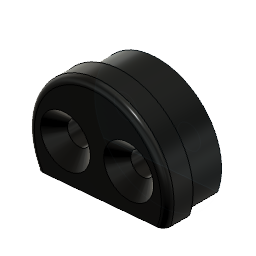
012_RVN_3DP_Shoulder_InnerShaft (Autodesk Fusion 360 design; units mm, degrees)
Autodesk Fusion 360 part; units mm, degrees
derive "DerivedContext1" from "RAVEN v69"
sketch "스케치1" plane through (0, 0, 0) normal (0, 0, 1) x (1, 0, 0)
  circle A0 centre (0, 0) radius 10
  circle A1 centre (0, 0) radius 11
  dimension "d1" = 20
  dimension "d2" = 22
  constraint coincident A0.centre A1.centre
  constraint concentric A0 A1
  measures "d1" diameter of A0
  measures "d2" diameter of A1
extrude "돌출1" add sketch "스케치1" against normal blind 7.5 contours A0
extrude "돌출2" add sketch "스케치1" along normal blind 2 contours A0 | A1
fillet "필렛1" radius 1 1 edges at (-10.2556, -3.9778, 2)
sketch "스케치4" plane through (0, 0, -7.5) normal (0, 0, -1) x (-1, 0, 0)
  circle A0 centre (0, 0) radius 10
  line L0 (38.7221, -7.7565) -> (-39.4804, -0.9282)
  circle A1 centre (-4.8644, 1.7709) radius 1.5
  circle A2 centre (5.0977, 0.9011) radius 1.5
  line L1 (-53.7248, -40.4802) -> (-43.0156, -41.4153)
  line L2 (35.1869, -48.2436) -> (45.8962, -49.1787)
  line L3 (-54.5947, -50.4423) -> (45.0263, -59.1408)
  circle A3 centre (29.9026, -20.9304) radius 1.5
  circle A4 centre (-33.0776, -15.4312) radius 1.5
  arc A5 (-19.3439, 34.1522) -> (-25.4868, 29.8494) centre (0, 0) ccw
  circle A6 centre (-20.9407, 29.8955) radius 1.5
  arc A7 (-36.7709, 13.7281) -> (-38.7108, 6.4833) centre (0, 0) ccw
  circle A8 centre (-35.2579, 9.4409) radius 1.5
  arc A9 (39.2487, -0.3238) -> (38.5937, 7.1476) centre (0, 0) ccw
  circle A10 centre (36.3606, 3.1874) radius 1.5
  arc A11 (30.2743, 24.9805) -> (24.9701, 30.2829) centre (0, 0) ccw
  circle A12 centre (25.805, 25.8138) radius 1.5
  line L4 (-43.0156, -41.4153) -> (-39.1012, 3.4142)
  arc A13 (-25.4868, 29.8494) -> (-36.7709, 13.7281) centre (0, 0) ccw
  arc A14 (38.5937, 7.1476) -> (30.2743, 24.9805) centre (0, 0) ccw
  arc A15 (39.1012, -3.4142) -> (39.2487, -0.3238) centre (0, 0) ccw
  arc A16 (24.9701, 30.2829) -> (-19.3439, 34.1522) centre (0, 0) ccw
  arc A17 (-38.7108, 6.4833) -> (-39.1012, 3.4142) centre (0, 0) ccw
  line L5 (39.1012, -3.4142) -> (35.1869, -48.2436)
  line L6 (-53.7248, -40.4802) -> (-54.5947, -50.4423)
  line L7 (45.8962, -49.1787) -> (45.0263, -59.1408)
  constraint coincident L5 L0.start
  constraint coincident L4 L0.end
extrude "돌출3" cut sketch "스케치4" against normal blind 31 contours A0 L0 | A0 L0 L1 L2 L3 L4 L5 L6 L7 | A1 | A2 picked at (-3.1566, -4.5316)
chamfer "챔퍼1" distance 2 angle 45 2 edges at (-3.6992, 0.3587, 2) (6.2629, 1.2285, 2)
extrude "돌출4" add 1 faces at (-0.1651, 4.8455, -7.5) along direction (0, 0, -1) blind 3
extrude "돌출5" cut 1 faces at (-0.1651, 4.8455, -10.5) along direction (0, 0, 1) blind 2
move_face "면 간격띄우기1" offset -0.2 2 faces at (7.4227, 6.701, -2.5) (-1.1182, 9.9373, -8.1667)
move_face "면 간격띄우기2" offset -0.3 4 faces at (-6.5958, 0.8263, -2.8333) (3.3718, 1.6216, -5.6667) (2.1114, 0.4452, 1.5556) (-3.9814, -1.9432, 1.5556)
extrude "돌출6" cut 1 faces at (-0.4178, 4.8911, -8.5) along direction (0, 0, 1) blind 1
extrude "돌출7" add 1 faces at (-0.9203, 10.5402, 0) along direction (0, 0, -1) blind 2
move_face "면 간격띄우기3" offset 0.2 1 faces at (-8.8189, -4.274, -5.6667)
sketch "스케치5" plane through (0, 0, -7.5) normal (0, 0, -1) x (-1, 0, 0)
  line L0 (-9.345, -3.5595) -> (8.5867, -5.1252)
  arc A0 (8.5867, -5.1252) -> (-9.345, -3.5595) centre (0, 0) ccw
  circle A1 centre (-4.8644, 1.7709) radius 1.8
  circle A2 centre (5.0977, 0.9011) radius 1.8
named bodies: "RVN_3DP_Shoulder_InnerShaft"
